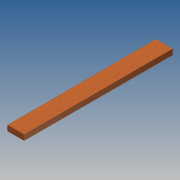
# Autodesk Inventor part: 1p2poscr
Saved by Autodesk Inventor 2014 SP1 (Build 180222100, 222)
## iProperties
Company: HERA Project
Created: 2014-04-30
Part Number: 1p2poscr
Material: Wood (Cherry)
Description: Pole screen holder
Document SubType Name: Modeling
Designer: Dave
Mass: 3794.01 g
Surface Area: 4143.54 cm^2
Volume: 6022.25 cm^3
Density: 0.63 g/cm^3
Appearance: Cherry - Natural Low Gloss
Title: Pole Screen Holder
Author: Dave
Autodesk Inventor part; units mm, degrees
ref_plane "YZ Plane" through (0, 0, 0) normal (1, 0, 0) x (0, 1, 0)
ref_plane "XZ Plane" through (0, 0, 0) normal (0, 1, 0) x (-1, 0, 0)
ref_plane "XY Plane" through (0, 0, 0) normal (0, 0, 1) x (1, 0, 0)
sketch "Sketch1" plane through (0, 0, 0) normal (0, 0, 1) x (1, 0, 0)
  line L0 (0, 0) -> (114, 0)
  line L1 (114, 0) -> (114, 38)
  line L2 (114, 38) -> (0, 38)
  line L3 (0, 38) -> (0, 0)
  dimension "d0" = 114
  dimension "d1" = 38
  constraints: 8 end point, 2 parallel, 1 horizontal, 1 perpendicular
  measures "d0" distance of L0.start L0.end
  measures "d1" distance of L2.end L0.start
extrude "Extrusion1" add sketch "Sketch1" along normal blind 1016
body "Solid1"
